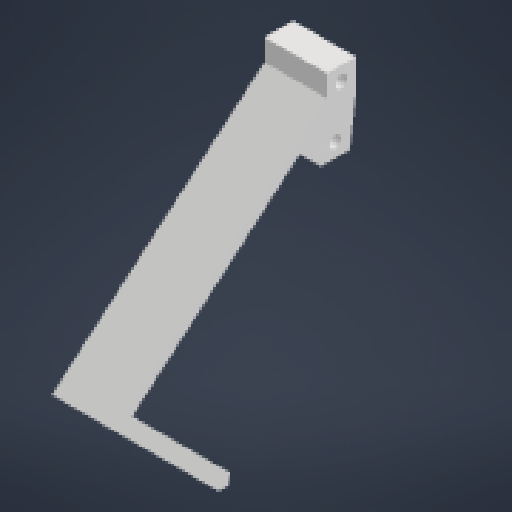
# Autodesk Inventor part: для ведра
Saved by Autodesk Inventor 2025 (Build 290162000, 162)
## iProperties
Created: 2025-03-17
Part Number: для ведра
Material: Типовые
Document SubType Name: Modeling
Designer: Phantom
Density: 1 g/cm^3
Appearance: По умолчанию
Author: Phantom
Autodesk Inventor part; units mm, degrees
ref_plane "YZ Plane" through (0, 0, 0) normal (1, 0, 0) x (0, 1, 0)
ref_plane "XZ Plane" through (0, 0, 0) normal (0, 1, 0) x (-1, 0, 0)
sketch "Эскиз1" plane through (0, 0, 0) normal (0, 0, 1) x (1, 0, 0)
  line L0 (0, 0) -> (58, 0)
  line L1 (58, 0) -> (58, 22)
  line L2 (58, 22) -> (0, 22)
  line L3 (0, 22) -> (0, 0)
  dimension "d8" = 58
  constraints: 8 end point, 2 parallel, 1 horizontal, 1 perpendicular
  measures "d8" distance of L0.start L0.end
extrude "Выдавливание1" add sketch "Эскиз1" along normal blind 3.2
sketch "Эскиз2" plane through (0, 0, 0) normal (-1, 0, 0) x (0, 0, 1)
  line L0 (-8.30128, 45.569732) -> (3.465123, -1.050454)
  line L1 (45.665123, 0) -> (-10.734877, 0)
  line L2 (3.465123, 39.725186) -> (31.465123, 39.725186)
  line L3 (31.465123, 39.725186) -> (31.465123, 9.630348)
  line L4 (31.465123, 9.630348) -> (3.465123, 9.630348)
  line L5 (3.465123, 9.630348) -> (3.465123, 39.725186)
  line L6 (-10.734877, 50.424514) -> (-10.734877, 0)
  line L7 (45.665123, 0) -> (-10.734877, 0)
  line L8 (45.665123, 50.424514) -> (45.665123, 0)
  line L9 (45.665123, 50.424514) -> (-10.734877, 50.424514)
  line L10 (3.2, 0) -> (3.2, 22)
  line L11 (0, 22) -> (0, 0)
  line L12 (0, 0) -> (3.2, 0)
  line L13 (3.2, 22) -> (3.2, 0)
  line L14 (0, 22) -> (3.2, 22)
  point P0 (17.465123, -2.237007)
  point P1 (3.2, 0)
  point P2 (0, 12.678862)
  point P3 (3.2, 0)
  constraints: 20 end point, 2 point on line
extrude "Выдавливание2" cut sketch "Эскиз2" against normal through all contours L11 L14 L10 L0
sketch "Эскиз3" plane through (0, 0, 0) normal (-1, 0, 0) x (0, 0, 1)
  line L0 (0, 12.678862) -> (0, 0)
  line L1 (3.2, 0) -> (0, 12.678862)
  line L2 (0, 12.678862) -> (0, 0)
  line L3 (0, 0) -> (3.2, 0)
  line L4 (3.2, 0) -> (-1.694295, 19.391902)
  line L5 (-1.694295, 19.391902) -> (-4.894295, 19.391902)
  line L6 (-4.894295, 19.391902) -> (0, 0)
  dimension "d4" = 20
  dimension "d5" = 3.2
  constraints: 6 end point, 1 horizontal
  measures "d4" distance of L1.start L4.end
  measures "d5" distance of L4.end L5.end
extrude "Выдавливание3" add sketch "Эскиз3" against normal blind 58 contours L0 L6 L5 L4
ref_plane "РабПлоскость1" through (21.759147, -32.255151, -128.653947) normal (-1, 0, 0) x (0, 0.0022468, 0.9999975)
sketch "Эскиз4" plane through (0, 19.391902, -4.894295) normal (-1, 0, 0) x (0, 0, 1)
  line L0 (8.094295, -19.391902) -> (3.2, 0)
  line L1 (3.2, 0) -> (0, 0)
  line L2 (0, 0) -> (4.894295, -19.391902)
  line L3 (4.894295, -19.391902) -> (8.094295, -19.391902)
  line L4 (-57.023054, -39.37846) -> (-64.753034, -39.395828)
  line L5 (-57.023054, -39.37846) -> (-57.060805, -22.576373)
  arc A0 (-52.262732, -21.586463) -> (-57.060805, -22.576373) centre (-54.560811, -22.570755) ccw
  line L6 (-52.262732, -21.586463) -> (-39.468155, -51.458617)
  line L7 (-39.468155, -51.458617) -> (-38.482965, -51.456404)
  line L8 (-38.500712, -43.55778) -> (-38.482965, -51.456404)
  line L9 (-38.500712, -43.55778) -> (-56.268061, -2.075439)
  arc A1 (-57.116102, 2.035) -> (-56.268061, -2.075439) centre (-46.616128, 2.058591) ccw
  line L10 (-57.116102, 2.035) -> (-57.215491, 46.270467)
  arc A2 (-57.215491, 46.270467) -> (-59.657453, 53.9842) centre (-70.715457, 46.240135) ccw
  line L11 (-59.657453, 53.9842) -> (-117.056864, 135.94669)
  arc A3 (-117.056864, 135.94669) -> (-119.842355, 136.437644) centre (-118.695086, 134.799421) ccw
  line L12 (-119.842355, 136.437644) -> (-122.897641, 134.297987)
  arc A4 (-122.897641, 134.297987) -> (-123.388595, 131.512495) centre (-121.750372, 132.659764) ccw
  line L13 (-123.388595, 131.512495) -> (-102.760997, 102.057675)
  arc A5 (-102.499562, 101.535947) -> (-102.760997, 102.057675) centre (-104.399219, 100.910406) ccw
  line L14 (-102.499562, 101.535947) -> (-64.912158, -12.610424)
  arc A6 (-64.81182, -13.231471) -> (-64.912158, -12.610424) centre (-66.811815, -13.235965) ccw
  line L15 (-64.81182, -13.231471) -> (-64.753034, -39.395828)
  circle A7 centre (-88.501405, 78.2094) radius 2.075
  circle A8 centre (-66.869679, 12.51763) radius 2.075
  circle A9 centre (-68.602336, 29.276127) radius 2.075
  circle A10 centre (-78.61848, 60.253701) radius 2.075
  circle A11 centre (-70.715457, 46.240135) radius 2.075
  circle A12 centre (-113.195156, 123.695864) radius 1.575
  circle A13 centre (-104.159361, 110.795596) radius 1.575
  circle A14 centre (-118.616633, 131.436024) radius 1.7325
  line L16 (-65.715457, 43.769729) -> (8.094295, -19.391902)
  line L17 (8.094295, -19.391902) -> (3.480151, -19.391902)
  line L18 (-56.199966, 31.678498) -> (3.480151, -19.391902)
  line L19 (-65.715457, 43.769729) -> (-65.715457, 51.240135)
  line L20 (-65.715457, 51.240135) -> (-75.715457, 51.240135)
  line L21 (-75.715457, 51.240135) -> (-75.715457, 41.240135)
  line L22 (-75.715457, 41.240135) -> (-65.715457, 51.240135) construction
  line L23 (-65.715457, 41.240135) -> (-72.282573, 47.807252) construction
  line L24 (-73.602336, 24.276127) -> (-63.602336, 24.276127)
  line L25 (-73.602336, 24.276127) -> (-63.602336, 34.276127) construction
  line L26 (-63.602336, 24.276127) -> (-73.602336, 34.276127) construction
  line L27 (-75.715457, 41.240135) -> (-73.602336, 24.276127)
  line L28 (-63.602336, 24.276127) -> (-56.199966, 31.678498)
  point P0 (4.012777, -15.899203)
  dimension "d10" = 3
  dimension "d11" = 10
  dimension "d12" = 10
  dimension "d13" = 10
  dimension "d14" = 10
  constraints: 26 end point, 3 midpoint, 2 horizontal, 2 parallel, 1 point on line, 1 other
  measures "d10" distance between parallel lines of L16 L18
  measures "d11" distance of L20.end L19.end
  measures "d12" distance of L19.end L23.start
  measures "d13" distance of L26.end L25.end
  measures "d14" distance of L25.end L24.end
extrude "Выдавливание4" add sketch "Эскиз4" against normal blind 20 contours L17 L18 L28 L10 L16 L2 | L10 L28 L24 L27 L21 L20 L19 L16
sketch "Эскиз5" plane through (0, 19.391902, -4.894295) normal (-1, 0, 0) x (0, 0, 1)
  circle A0 centre (-68.602336, 29.276127) radius 2.075
  circle A1 centre (-70.715457, 46.240135) radius 2.075
  line L0 (8.094295, -19.391902) -> (3.2, 0)
  line L1 (3.2, 0) -> (0, 0)
  line L2 (0, 0) -> (4.012777, -15.899203)
  line L3 (4.012777, -15.899203) -> (-65.715457, 43.769729)
  line L4 (-65.715457, 43.769729) -> (-65.715457, 51.240135)
  line L5 (-65.715457, 51.240135) -> (-75.715457, 51.240135)
  line L6 (-75.715457, 51.240135) -> (-75.715457, 41.240135)
  line L7 (-75.715457, 41.240135) -> (-73.602336, 24.276127)
  line L8 (-73.602336, 24.276127) -> (-63.602336, 24.276127)
  line L9 (-63.602336, 24.276127) -> (-56.199966, 31.678498)
  line L10 (-56.199966, 31.678498) -> (3.480151, -19.391902)
  line L11 (3.480151, -19.391902) -> (8.094295, -19.391902)
  line L12 (4.012777, -15.899203) -> (28.670858, -37)
  point P0 (4.894295, -19.391902)
  constraints: 2 end point
extrude "Выдавливание5" cut sketch "Эскиз5" against normal through all contours L12 L2 L1 L0
sketch "Эскиз6" plane through (21.759147, 60.632037, -80.609751) normal (1, 0, 0) x (0, 0, -1)
  line L0 (-79.195607, -60.632037) -> (-19.515491, -9.561637)
  line L1 (-19.515491, -9.561637) -> (-12.11312, -16.964007)
  line L2 (-12.11312, -16.964007) -> (-2.11312, -16.964007)
  line L3 (-2.11312, -16.964007) -> (0, 0)
  line L4 (0, 0) -> (0, 10)
  line L5 (0, 10) -> (-10, 10)
  line L6 (-10, 10) -> (-10, 2.529594)
  line L7 (-10, 2.529594) -> (-79.728234, -57.139337)
  line L8 (-80.609751, -60.632037) -> (-79.728234, -57.139337)
  line L9 (-80.609751, -60.632037) -> (-79.195607, -60.632037)
  circle A0 centre (-5, 5) radius 2.075
  circle A1 centre (-7.11312, -11.964007) radius 2.075
  line L10 (-19.515491, -9.561637) -> (-19.515491, 2.529594)
  point P0 (-80.609751, -60.632037)
  point P1 (-19.515491, -5.61315)
  constraints: 2 end point, 1 vertical
extrude "Выдавливание6" [suppressed]
sketch "Эскиз7" plane through (58, 0, 3.2) normal (1, 0, 0) x (0, 0, -1)
  circle A0 centre (76.696631, 48.66803) radius 2.075
  line L0 (0, 0) -> (73.809751, 63.161631)
  line L1 (73.809751, 63.161631) -> (73.809751, 70.632037)
  line L2 (73.809751, 70.632037) -> (83.809751, 70.632037)
  line L3 (83.809751, 70.632037) -> (83.809751, 60.632037)
  line L4 (83.809751, 60.632037) -> (81.696631, 43.66803)
  line L5 (81.696631, 43.66803) -> (71.696631, 43.66803)
  line L6 (71.696631, 43.66803) -> (64.294261, 51.0704)
  line L7 (64.294261, 51.0704) -> (4.614144, 0)
  line L8 (4.614144, 0) -> (0, 0)
  circle A1 centre (78.809751, 65.632037) radius 2.075
  circle A2 centre (76.696631, 48.66803) radius 2.075
  line L9 (64.294261, 55.018887) -> (64.294261, 51.0704)
  point P0 (3.2, 0)
extrude "Выдавливание7" add sketch "Эскиз7" against normal blind 18 contours L0 L1 L2 L3 L4 L5 L6 L9
sketch "Эскиз8" plane through (20, 19.391902, -4.894295) normal (1, 0, 0) x (0, 0, -1)
  line L0 (56.199966, 31.678498) -> (63.602336, 24.276127)
  line L1 (63.602336, 24.276127) -> (73.602336, 24.276127)
  line L2 (73.602336, 24.276127) -> (75.715457, 41.240135)
  line L3 (75.715457, 41.240135) -> (75.715457, 51.240135)
  line L4 (75.715457, 51.240135) -> (65.715457, 51.240135)
  line L5 (65.715457, 51.240135) -> (65.715457, 43.769729)
  line L6 (65.715457, 43.769729) -> (-4.012777, -15.899203)
  line L7 (-4.894295, -19.391902) -> (-4.012777, -15.899203)
  line L8 (-4.894295, -19.391902) -> (-3.480151, -19.391902)
  line L9 (-3.480151, -19.391902) -> (56.199966, 31.678498)
  circle A0 centre (70.715457, 46.240135) radius 2.075
  circle A1 centre (68.602336, 29.276127) radius 2.075
  line L10 (56.199966, 31.678498) -> (56.199966, 44.165135)
  point P0 (56.199966, 35.626985)
  constraints: 2 end point, 1 vertical
extrude "Выдавливание8" add sketch "Эскиз8" along normal up to surface (38 mm away) contours L9 L8 L7 L6 L10
sketch "Эскиз9" plane through (58, 0, 3.2) normal (1, 0, 0) x (0, 0, -1)
  circle A0 centre (76.696631, 48.66803) radius 2.075
  circle A1 centre (78.809751, 65.632037) radius 2.075
  line L0 (73.809751, 63.161631) -> (0, 0)
  line L1 (4.614144, 0) -> (0, 0)
  line L2 (64.294261, 51.0704) -> (4.614144, 0)
  line L3 (64.294261, 51.0704) -> (71.696631, 43.66803)
  line L4 (71.696631, 43.66803) -> (81.696631, 43.66803)
  line L5 (81.696631, 43.66803) -> (83.809751, 60.632037)
  line L6 (83.809751, 60.632037) -> (83.809751, 70.632037)
  line L7 (83.809751, 70.632037) -> (73.809751, 70.632037)
  line L8 (73.809751, 70.632037) -> (73.809751, 63.161631)
  line L9 (64.294261, 51.0704) -> (64.294261, 61)
  point P0 (3.2, 0)
  point P1 (64.294261, 55.018887)
  constraints: 2 end point, 1 vertical
extrude "Выдавливание9" cut sketch "Эскиз9" against normal blind 10 contours L8 L7 L6 L5 L4 L3 L9 L0
sketch "Эскиз10" plane through (0, 60.632037, -80.609751) normal (-1, 0, 0) x (0, 0, 1)
  line L0 (83.809751, -60.632037) -> (10, 2.529594)
  line L1 (10, 2.529594) -> (10, 10)
  line L2 (10, 10) -> (0, 10)
  line L3 (0, 10) -> (0, 0)
  line L4 (0, 0) -> (2.11312, -16.964007)
  line L5 (2.11312, -16.964007) -> (12.11312, -16.964007)
  line L6 (12.11312, -16.964007) -> (19.515491, -9.561637)
  line L7 (19.515491, -9.561637) -> (79.195607, -60.632037)
  line L8 (79.195607, -60.632037) -> (83.809751, -60.632037)
  circle A0 centre (5, 5) radius 2.075
  circle A1 centre (7.11312, -11.964007) radius 2.075
  line L9 (19.515491, -9.561637) -> (19.515491, 20)
  point P0 (80.609751, -60.632037)
  point P1 (19.515491, -5.61315)
  constraints: 2 end point, 1 vertical
extrude "Выдавливание10" cut sketch "Эскиз10" against normal blind 10 contours L9 L6 L5 L4 L3 L2 L1 L0
fillet "Сопряжение1" radius 9 2 edges at (0, 53.0446, -61.0943) (58, 53.0446, -61.0943)
fillet "Сопряжение2" radius 9 2 edges at (10, 53.0446, -61.0943) (48, 53.0446, -61.0943)
fillet "Сопряжение3" radius 6 6 edges at (15, 51.0704, -61.0943) (15, 43.668, -68.4966) (15, 43.668, -78.4966) (44, 43.668, -78.4966) (44, 43.668, -68.4966) (44, 51.0704, -61.0943)
fillet "Сопряжение4" radius 4 4 edges at (15, 70.632, -70.6098) (15, 70.632, -80.6098) (44, 70.632, -70.6098) (44, 70.632, -80.6098)
sketch "Эскиз11" plane through (0, 0, -1.414144) normal (-1, 0, 0) x (0, 0, 1)
  line L0 (-50.680117, 43.36878) -> (0, 0)
  line L1 (-71.783507, 43.66803) -> (0, 0)
  line L2 (-71.783507, 43.66803) -> (-69.662186, 45.78935)
  line L3 (-63.605737, 47.144781) -> (-65.325128, 45.425389)
  line L4 (-69.662186, 45.78935) -> (-13.790215, 11.800778)
  point P0 (1.414144, 0)
  dimension "d33" = 3
  constraints: 6 end point, 2 parallel, 1 point on line
  measures "d33" distance of L1.start L2.end
extrude "Выдавливание11" add sketch "Эскиз11" against normal up to surface (20 mm away)
sketch "Эскиз12" plane through (0, 43.36878, -52.094261) normal (-1, 0, 0) x (0, 0, 1)
  line L0 (-21.10339, 0.29925) -> (50.680117, -43.36878)
  line L1 (0, 0) -> (0, 3.948487)
  line L2 (0, 0) -> (36.889902, -31.568002)
  line L3 (36.889902, -31.568002) -> (-18.982069, 2.42057)
  line L4 (-18.982069, 2.42057) -> (-21.10339, 0.29925)
  line L5 (-21.10339, 0.29925) -> (50.680117, -43.36878)
  line L6 (50.680117, -43.36878) -> (55.294261, -43.36878)
  line L7 (55.294261, -43.36878) -> (0, 3.948487)
  line L8 (36.889902, -31.568002) -> (50.680117, -43.36878)
  point P0 (52.094261, -43.36878)
  constraints: 2 end point
extrude "Выдавливание12" cut sketch "Эскиз12" against normal up to surface (10 mm away) contours L4 L3 L8 L0
sketch "Эскиз13" plane through (48, 0, 3.2) normal (1, 0, 0) x (0, 0, -1)
  arc A0 (76.397651, 43.66803) -> (82.351636, 48.926372) centre (76.397651, 49.66803) ccw
  line L0 (82.351636, 48.926372) -> (83.809751, 60.632037)
  line L1 (83.809751, 60.632037) -> (83.809751, 66.632037)
  arc A1 (83.809751, 66.632037) -> (79.809751, 70.632037) centre (79.809751, 66.632037) ccw
  line L2 (79.809751, 70.632037) -> (77.809751, 70.632037)
  arc A2 (77.809751, 70.632037) -> (73.809751, 66.632037) centre (77.809751, 66.632037) ccw
  line L3 (73.809751, 66.632037) -> (73.809751, 63.161631)
  line L4 (73.809751, 63.161631) -> (64.294261, 55.018887)
  line L5 (64.294261, 55.018887) -> (64.294261, 48.893759)
  arc A3 (68.21988, 47.144781) -> (64.294261, 48.893759) centre (63.97724, 42.90214) ccw
  line L6 (68.21988, 47.144781) -> (69.939272, 45.425389)
  arc A4 (69.939272, 45.425389) -> (71.684336, 44.212564) centre (74.181912, 49.66803) ccw
  line L7 (71.684336, 44.212564) -> (18.404359, 11.800778)
  line L8 (4.614144, 0) -> (18.404359, 11.800778)
  line L9 (4.614144, 0) -> (76.397651, 43.66803)
  circle A5 centre (78.809751, 65.632037) radius 2.075
  circle A6 centre (76.696631, 48.66803) radius 2.075
  circle A7 centre (76.696631, 48.66803) radius 2.075
  circle A8 centre (78.809751, 65.632037) radius 2.075
  arc A9 (83.809751, 66.632037) -> (79.809751, 70.632037) centre (79.809751, 66.632037) ccw
  line L10 (77.809751, 70.632037) -> (79.809751, 70.632037)
  arc A10 (77.809751, 70.632037) -> (73.809751, 66.632037) centre (77.809751, 66.632037) ccw
  line L11 (73.809751, 63.161631) -> (73.809751, 66.632037)
  line L12 (71.418776, 61.115589) -> (73.809751, 63.161631)
  line L13 (71.418776, 57.167102) -> (71.418776, 61.115589)
  line L14 (71.418776, 57.167102) -> (64.294261, 51.0704)
  line L15 (64.294261, 48.893759) -> (64.294261, 51.0704)
  arc A11 (68.21988, 47.144781) -> (64.294261, 48.893759) centre (63.97724, 42.90214) ccw
  line L16 (69.939272, 45.425389) -> (68.21988, 47.144781)
  arc A12 (69.939272, 45.425389) -> (74.181912, 43.66803) centre (74.181912, 49.66803) ccw
  line L17 (76.397651, 43.66803) -> (74.181912, 43.66803)
  arc A13 (76.397651, 43.66803) -> (82.351636, 48.926372) centre (76.397651, 49.66803) ccw
  line L18 (83.809751, 60.632037) -> (82.351636, 48.926372)
  line L19 (83.809751, 66.632037) -> (83.809751, 60.632037)
  point P0 (3.2, 0)
  point P1 (71.684336, 44.212564)
extrude "Выдавливание13" add sketch "Эскиз13" against normal up to surface (8 mm away) contours L9 L8 L7 A12 L17
